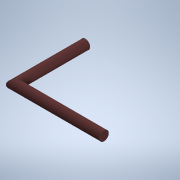
# Autodesk Inventor part: palanca
Saved by Autodesk Inventor 2021.1 (Build 251245000, 245)
## iProperties
Created: 2021-01-01
Part Number: palanca
Material: Generic
Document SubType Name: Modeling
Designer: Bolisteward
Density: 1 g/cm^3
Appearance: Default
Author: Bolisteward
Autodesk Inventor part; units mm, degrees
ref_plane "YZ Plane" through (0, 0, 0) normal (1, 0, 0) x (0, 1, 0)
ref_plane "XZ Plane" through (0, 0, 0) normal (0, 1, 0) x (-1, 0, 0)
ref_plane "XY Plane" through (0, 0, 0) normal (0, 0, 1) x (1, 0, 0)
sketch "Sketch1" plane through (0, 0, 0) normal (0, 1, 0) x (-1, 0, 0)
  line L0 (0, 0) -> (50, 0)
  line L1 (50, 0) -> (50, -5)
  line L2 (50, -5) -> (0, -5)
  line L3 (0, -5) -> (0, 0)
  line L4 (50, 0) -> (45, 0)
  line L5 (45, 0) -> (45, -40)
  line L6 (45, -40) -> (50, -40)
  line L7 (50, -40) -> (50, 0)
  point P0 (45, -5)
  dimension "d0" = 50
  dimension "d1" = 5
  dimension "d2" = 5
  dimension "d3" = 40
  constraints: 16 end point, 4 parallel, 2 horizontal, 2 perpendicular
  measures "d0" distance of L1.end L2.end
  measures "d1" distance of L0.end L1.end
  measures "d2" distance of L6.end L5.end
  measures "d3" distance of L5.end L4.end
extrude "Extrusion1" add sketch "Sketch1" along normal blind 5
fillet "Fillet1" radius 2.5 10 edges at (-25, 5, 0) (-50, 5, -2.5) (-50, 5, -22.5) (-25, 0, 0) (-50, 0, -2.5) (-50, 0, -22.5) (-45, 0, -22.5) (-45, 5, -22.5) (-22.5, 5, -5) (-22.5, 0, -5)
body "Solid1"
